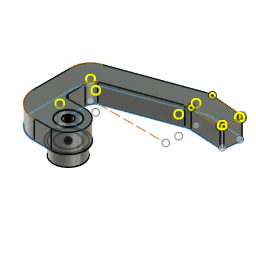
uselessbox-arm (Autodesk Fusion 360 design; units mm, degrees)
Autodesk Fusion 360 part; units mm, degrees
sketch "Sketch1" plane through (0, 0, 0) normal (0, 0, 1) x (1, 0, 0)
  circle A0 centre (0, 0) radius 2.45
  circle A1 centre (0, 0) radius 3.5
  circle A2 centre (0, 0) radius 4
  line L0 (0, 4) -> (-4, 4)
  arc A3 (-5, 5) -> (-4, 4) centre (-4, 5) ccw
  line L1 (-5, 5) -> (-5, 9)
  line L2 (-4, 11) -> (11.0351, 16.4723)
  line L3 (-4, 11) -> (12, 11) construction
  line L4 (0, -4) -> (-4, -4)
  line L5 (-10, 1.5) -> (-10, 10.4947)
  line L6 (-7, 15) -> (11.2229, 21.6326)
  arc A4 (-10, 1.5) -> (-4, -4) centre (-4, 2.0227) ccw
  arc A5 (-4, 11) -> (-5, 9) centre (-2.5, 9) ccw
  arc A6 (-7, 15) -> (-10, 10.4947) centre (-5.438, 10.7084) ccw
  line L7 (12.3, 16.7) -> (19.5014, 16.3173)
  line L8 (12.3, 21.7) -> (20, 21)
  line L9 (20, 16.7) -> (20.5, 20.5)
  arc A7 (20.5, 20.5) -> (20, 21) centre (19.95, 20.45) ccw
  arc A8 (19.5014, 16.3173) -> (20, 16.7) centre (19.527, 16.8001) ccw
  arc A9 (12.3, 21.7) -> (11.2229, 21.6326) centre (11.9798, 18.1776) ccw
  arc A10 (12.3, 16.7) -> (11.0351, 16.4723) centre (12.1512, 13.8992) ccw
  dimension "d1" = 4.9
  dimension "d2" = 7
  dimension "d3" = 8
  dimension "d4" = 4
  dimension "d6" = 20
  dimension "d7" = 16
  constraint coincident A0.centre A1.centre
  constraint concentric A0 A1
  constraint coincident A2 L0.start
  constraint horizontal L0
  constraint vertical L1
  constraint horizontal L3
  constraint coincident A2 L4.start
  constraint horizontal L4
  constraint vertical L5
  constraint parallel L2 L6
  constraint tangent L4 A4
  constraint tangent L1 A5
  constraint tangent L6 A6
  constraint tangent L8 A7
  constraint tangent L7 A8
  constraint tangent L8 A9
  constraint tangent L7 A10
  measures "d1" diameter of A0
  measures "d2" diameter of A1
  measures "d3" diameter of A2
  measures "d4" distance of L0.start L0.end
  measures "d6" angle of L2 L3
  measures "d7" distance of L2.start L2.end
sketch "Sketch2" plane through (0, 0, 4.5) normal (0, 0, 1) x (-1, 0, 0)
  line L0 (10, -10.4947) -> (10, -1.5)
  line L1 (4, 4) -> (0, 4)
  arc A0 (0, 4) -> (0, -4) centre (0, 0) ccw
  line L2 (0, -4) -> (4, -4)
  arc A1 (5, -5) -> (4, -4) centre (4, -5) ccw
  line L3 (5, -5) -> (5, -9)
  line L4 (4, -11) -> (-11.0351, -16.4723)
  line L5 (-11.2229, -21.6326) -> (7, -15)
  circle A2 centre (0, 0) radius 2.5
  circle A3 centre (0, 0) radius 1.1
  arc A4 (4, -11) -> (5, -9) centre (2.5, -9) ccw
  arc A5 (-12.3, -16.7) -> (-11.0351, -16.4723) centre (-12.1512, -13.8992) ccw
  line L6 (-12.3, -16.7) -> (-19.5014, -16.3173)
  arc A6 (-19.5014, -16.3173) -> (-20, -16.7) centre (-19.527, -16.8001) ccw
  line L7 (-20, -16.7) -> (-20.5, -20.5)
  arc A7 (-20.5, -20.5) -> (-20, -21) centre (-19.95, -20.45) ccw
  line L8 (-20, -21) -> (-12.3, -21.7)
  arc A8 (-12.3, -21.7) -> (-11.2229, -21.6326) centre (-11.9798, -18.1776) ccw
  arc A9 (7, -15) -> (10, -10.4947) centre (5.438, -10.7084) ccw
  arc A10 (10, -1.5) -> (4, 4) centre (4, -2.0227) ccw
  dimension "d14" = 5
  dimension "d15" = 2.2
  constraint concentric A0 A2
  constraint concentric A0 A3
  measures "d14" diameter of A2
  measures "d15" diameter of A3
extrude "Extrude5" add sketch "Sketch1" along normal blind 4.5 contours A0 | A1 | A2 | A2 L0 A3 L1 L2 L4 L5 L6 A4 A5 A6 L7 L8 L9 A7 A8 A9 A10
extrude "Extrude6" cut sketch "Sketch2" against normal blind 3.5 contours A2
extrude "Extrude7" cut sketch "Sketch2" against normal blind 5 contours A3
extrude "Extrude8" add sketch "Sketch1" against normal blind 3 contours A1
